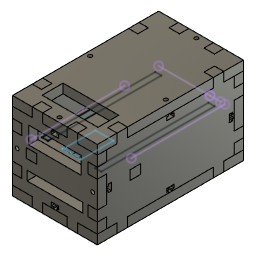
Basic-Case (Autodesk Fusion 360 design; units mm, degrees)
Autodesk Fusion 360 part; units mm, degrees
(part 1 of 2)
ref_plane "WorkPlane4" through (0, 29.5, 0) normal (0, 1, 0) x (0, 0, 1)
ref_plane "WorkPlane5" through (0, 0, 27.5) normal (0, 0, 1) x (1, 0, 0)
ref_plane "WorkPlane9" through (0, 0, -27.5) normal (0, 0, 1) x (1, 0, 0)
ref_plane "WorkPlane11" through (-14.285, 0, 0) normal (1, 0, 0) x (0, 1, 0)
ref_plane "WorkPlane12" through (14.285, 0, 0) normal (1, 0, 0) x (0, 1, 0)
sketch "Sketch1" plane through (0, 0, 0) normal (0, 1, 0) x (1, 0, 0)
  line L0 (12.785, -26) -> (-12.785, -26) construction
  line L1 (-12.785, -26) -> (-12.785, 26) construction
  line L2 (-12.785, 26) -> (12.785, 26) construction
  line L3 (12.785, 26) -> (12.785, -26) construction
  line L4 (12.785, -26) -> (-12.785, 26) construction
  line L5 (-12.785, -26) -> (12.785, 26) construction
  line L6 (-14.285, -27.5) -> (-14.285, 27.5)
  line L7 (-14.285, 27.5) -> (14.285, 27.5)
  line L8 (14.285, 27.5) -> (14.285, -27.5)
  line L9 (14.285, -27.5) -> (-14.285, -27.5)
  line L10 (-18.285, -31.5) -> (-18.285, 31.5)
  line L11 (-18.285, 31.5) -> (18.285, 31.5)
  line L12 (18.285, 31.5) -> (18.285, -31.5)
  line L13 (18.285, -31.5) -> (-18.285, -31.5)
  line L14 (-18.285, -23) -> (-12.785, -23)
  line L15 (-18.285, -18.5) -> (-14.285, -18.5)
  line L16 (-9.785, -27.5) -> (-9.785, -31.5)
  line L17 (-5.285, -31.5) -> (-5.285, -27.5)
  line L18 (5.285, -27.5) -> (5.285, -31.5)
  line L19 (9.785, -31.5) -> (9.785, -27.5)
  line L20 (14.285, -23) -> (18.285, -23)
  line L21 (14.285, -18.5) -> (18.285, -18.5)
  line L22 (14.285, 23) -> (18.285, 23)
  line L23 (18.285, 18.5) -> (14.285, 18.5)
  line L24 (9.785, 31.5) -> (9.785, 27.5)
  line L25 (5.285, 31.5) -> (5.285, 27.5)
  line L26 (-9.785, 31.5) -> (-9.785, 27.5)
  line L27 (-5.285, 27.5) -> (-5.285, 31.5)
  line L28 (-14.285, 23) -> (-18.285, 23)
  line L29 (-18.285, 18.5) -> (-14.285, 18.5)
  line L30 (0, -27.5) -> (0, -31.5) construction
  line L31 (14.285, 0) -> (18.285, 0) construction
  line L32 (-18.285, 0) -> (-14.285, 0) construction
  line L33 (0, 31.5) -> (0, 27.5) construction
  circle A0 centre (16.285, 0) radius 0.8
  circle A1 centre (0, 29.5) radius 0.8
  circle A2 centre (-16.285, 0) radius 0.8
  circle A3 centre (0, -29.5) radius 0.8
  dimension "d1" = 52
  dimension "d2" = 25.57
  dimension "d3" = 1.5
  dimension "d4" = 5.5
  dimension "d385" = 4.5
  dimension "d386" = 4.5
  dimension "d387" = 4.5
  dimension "d388" = 4.5
  dimension "d389" = 4.5
  dimension "d391" = 4.5
  dimension "d392" = 4.5
  dimension "d394" = 4.5
  dimension "d395" = 4.5
  dimension "d396" = 4.5
  dimension "d397" = 4.5
  dimension "d399" = 4.5
  dimension "d402" = 1.6
  dimension "d403" = 1.6
  dimension "d404" = 1.6
  dimension "d405" = 1.6
  dimension "d437" = 4.5
  dimension "d438" = 4.5
  dimension "d439" = 4.5
  dimension "d440" = 4.5
  constraint perpendicular L0 L1
  constraint parallel L0 L2
  constraint parallel L1 L3
  constraint horizontal L0
  constraint coincident L4 origin
  constraint coincident L5 origin
  constraint coincident L10 L14.start
  constraint coincident L1 L14.end
  constraint perpendicular L6 L14
  constraint coincident L10 L15.start
  constraint coincident L6 L15.end
  constraint perpendicular L1 L15
  constraint coincident L9 L16.start
  constraint coincident L13 L16.end
  constraint perpendicular L13 L16
  constraint coincident L13 L17.start
  constraint coincident L9 L17.end
  constraint perpendicular L9 L17
  constraint coincident L9 L18.start
  constraint coincident L13 L18.end
  constraint perpendicular L13 L18
  constraint coincident L13 L19.start
  constraint coincident L9 L19.end
  constraint perpendicular L0 L19
  constraint coincident L8 L20.start
  constraint coincident L12 L20.end
  constraint perpendicular L12 L20
  constraint coincident L8 L21.start
  constraint coincident L12 L21.end
  constraint perpendicular L12 L21
  constraint coincident L8 L22.start
  constraint coincident L12 L22.end
  constraint perpendicular L12 L22
  constraint coincident L12 L23.start
  constraint coincident L8 L23.end
  constraint perpendicular L8 L23
  constraint coincident L11 L24.start
  constraint coincident L7 L24.end
  constraint perpendicular L7 L24
  constraint coincident L11 L25.start
  constraint coincident L7 L25.end
  constraint perpendicular L11 L25
  constraint coincident L11 L26.start
  constraint coincident L7 L26.end
  constraint perpendicular L7 L26
  constraint coincident L7 L27.start
  constraint coincident L11 L27.end
  constraint perpendicular L11 L27
  constraint coincident L6 L28.start
  constraint coincident L10 L28.end
  constraint perpendicular L10 L28
  constraint coincident L10 L29.start
  constraint coincident L6 L29.end
  constraint perpendicular L6 L29
  constraint midpoint L9 L30.start
  constraint midpoint L13 L30.end
  constraint midpoint L8 L31.start
  constraint midpoint L12 L31.end
  constraint midpoint L10 L32.start
  constraint midpoint L6 L32.end
  constraint midpoint L11 L33.start
  constraint midpoint L7 L33.end
  constraint midpoint L31 A0.centre
  constraint midpoint L33 A1.centre
  constraint midpoint L32 A2.centre
  constraint midpoint L30 A3.centre
  measures "d1" distance of L0.start L2.end
  measures "d2" distance of L0.start L0.end
  measures "d385" distance of L28 L29
  measures "d386" distance of L26 L27
  measures "d387" distance of L6.end L26
  measures "d388" distance of L24 L25
  measures "d389" distance of L7.end L24
  measures "d391" distance of L22 L23
  measures "d392" distance of L20 L21
  measures "d394" distance of L8.end L19
  measures "d395" distance of L18 L19
  measures "d396" distance of L6.start L16
  measures "d397" distance of L16 L17
  measures "d399" distance of L14 L15
  measures "d402" diameter of A3
  measures "d403" diameter of A0
  measures "d404" diameter of A2
  measures "d405" diameter of A1
  measures "d437" distance of L6.start L14
  measures "d438" distance of L6.end L28
  measures "d439" distance of L7.end L22
  measures "d440" distance of L8.end L20
sketch "Sketch33" plane through (0, 29.5, 0) normal (0, 1, 0) x (1, 0, 0)
  line L0 (-18.285, 31.5) -> (18.285, 31.5)
  line L1 (-18.285, -31.5) -> (-18.285, 31.5)
  line L2 (18.285, -31.5) -> (-18.285, -31.5)
  line L3 (-14.285, -27.5) -> (-14.285, 27.5)
  line L4 (-14.285, 27.5) -> (14.285, 27.5)
  line L5 (-14.285, 23) -> (-18.285, 23)
  line L6 (-18.285, 18.5) -> (-14.285, 18.5)
  line L7 (-9.785, 31.5) -> (-9.785, 27.5)
  line L8 (-5.285, 27.5) -> (-5.285, 31.5)
  line L9 (5.285, 31.5) -> (5.285, 27.5)
  line L10 (9.785, 31.5) -> (9.785, 27.5)
  line L11 (14.285, 27.5) -> (14.285, -27.5)
  line L12 (14.285, 23) -> (18.285, 23)
  line L13 (18.285, 18.5) -> (14.285, 18.5)
  line L14 (18.285, 31.5) -> (18.285, -31.5)
  line L15 (14.285, -18.5) -> (18.285, -18.5)
  line L16 (14.285, -23) -> (18.285, -23)
  line L17 (9.785, -31.5) -> (9.785, -27.5)
  line L18 (5.285, -27.5) -> (5.285, -31.5)
  line L19 (-5.285, -31.5) -> (-5.285, -27.5)
  line L20 (-9.785, -27.5) -> (-9.785, -31.5)
  line L21 (-18.285, -23) -> (-12.785, -23)
  line L22 (-18.285, -18.5) -> (-14.285, -18.5)
  line L23 (14.285, -27.5) -> (-14.285, -27.5)
  circle A0 centre (0, -29.5) radius 0.8
  circle A1 centre (0, 29.5) radius 0.8
  circle A2 centre (-16.285, 0) radius 0.8
  circle A3 centre (16.285, 0) radius 0.8
  point P0 (16.285, 0)
  point P1 (-16.285, 0)
sketch "Sketch24" plane through (0, 0, 27.5) normal (0, 0, 1) x (1, 0, 0)
  line L0 (18.285, 0) -> (-18.285, 0)
  line L1 (18.285, 29.5) -> (-18.285, 29.5)
  line L2 (-9.785, 29.5) -> (-9.785, 33.5)
  line L3 (-5.285, 29.5) -> (-5.285, 33.5)
  line L4 (5.285, 29.5) -> (5.285, 33.5)
  line L5 (9.785, 29.5) -> (9.785, 33.5)
  line L6 (-9.785, 0) -> (-9.785, -4)
  line L7 (-5.285, 0) -> (-5.285, -4)
  line L8 (5.285, 0) -> (5.285, -4)
  line L9 (9.785, 0) -> (9.785, -4)
  line L10 (-0.8, 29.5) -> (-0.8, 28.8)
  line L11 (-0.8, 28.8) -> (-1.6, 28.8)
  line L12 (-1.6, 28.8) -> (-1.6, 27.4)
  line L13 (-1.6, 27.4) -> (1.6, 27.4)
  line L14 (1.6, 27.4) -> (1.6, 28.8)
  line L15 (1.6, 28.8) -> (0.8, 28.8)
  line L16 (0.8, 28.8) -> (0.8, 29.5)
  line L17 (-0.8, 0) -> (-0.8, 0.7)
  line L18 (-1.6, 0.7) -> (-1.6, 2.1)
  line L19 (-1.6, 2.1) -> (1.6, 2.1)
  line L20 (-0.8, 0.7) -> (-1.6, 0.7)
  line L21 (1.6, 0.7) -> (0.8, 0.7)
  line L22 (0.8, 0.7) -> (0.8, 0)
  line L23 (1.6, 2.1) -> (1.6, 0.7)
  line L24 (0, 27.4) -> (0, 29.5) construction
  line L25 (0, 2.1) -> (0, 0) construction
  line L26 (14.285, 25) -> (24.3607, 25)
  line L27 (14.285, 4.5) -> (18.285, 4.5)
  line L28 (-14.285, 20.5) -> (-18.285, 20.5)
  line L29 (-18.285, 9) -> (-14.285, 9)
  line L30 (-18.285, 33.5) -> (-18.285, -4)
  line L31 (-18.285, -4) -> (18.285, -4)
  line L32 (18.285, -4) -> (18.285, 33.5)
  line L33 (18.285, 33.5) -> (-18.285, 33.5)
  line L34 (-14.285, 29.5) -> (-14.285, 0)
  line L35 (14.285, 29.5) -> (14.285, 0)
  line L36 (18.285, 9) -> (14.285, 9)
  line L37 (18.285, 20.5) -> (14.285, 20.5)
  line L38 (-14.285, 25) -> (-18.285, 25)
  line L39 (-14.285, 4.5) -> (-18.285, 4.5)
  line L40 (18.285, 14.75) -> (14.285, 14.75) construction
  line L41 (-14.285, 14.75) -> (-14.285, 14.6467)
  line L42 (-18.285, 14.75) -> (-14.285, 14.75) construction
  circle A0 centre (16.285, 14.75) radius 0.8
  circle A1 centre (-16.285, 14.75) radius 0.8
  line L43 (0, 0) -> (0, 33.5) construction
  point P0 (-5.285, 0)
  point P1 (-9.785, 0)
  point P2 (5.285, 0)
  point P3 (9.785, 0)
  point P4 (0, 29.5)
  point P5 (-9.785, 29.5)
  point P6 (-5.285, 29.5)
  point P7 (9.785, 29.5)
  point P8 (5.285, 29.5)
  dimension "d406" = 3.2
  dimension "d407" = 1.4
  dimension "d409" = 1.6
  dimension "d410" = 1.6
  dimension "d411" = 3.2
  dimension "d413" = 1.4
  dimension "d420" = 6.1
  dimension "d421" = 4
  dimension "d422" = 4
  dimension "d424" = 6.1
  dimension "d425" = 4
  dimension "d426" = 4
  dimension "d427" = 4.5
  dimension "d428" = 4.5
  dimension "d429" = 4.5
  dimension "d430" = 4.5
  dimension "d433" = 4.5
  dimension "d434" = 4.5
  dimension "d435" = 1.6
  dimension "d436" = 1.6
  dimension "d482" = 4.5
  dimension "d483" = 4.5
  constraint coincident P1 L6.start
  constraint coincident P0 L7.start
  constraint coincident P2 L8.start
  constraint perpendicular L0 L8
  constraint coincident P3 L9.start
  constraint perpendicular L10 L11
  constraint perpendicular L12 L13
  constraint perpendicular L14 L15
  constraint collinear L11 L15
  constraint equal L11 L15
  constraint equal L17 L22
  constraint equal L18 L23
  constraint equal L20 L21
  constraint perpendicular L18 L19
  constraint perpendicular L19 L23
  constraint perpendicular L18 L20
  constraint perpendicular L21 L22
  constraint midpoint L13 L24.start
  constraint coincident P4 L24.end
  constraint perpendicular L1 L24
  constraint midpoint L19 L25.start
  constraint coincident L25.end L43.start
  constraint perpendicular L0 L25
  constraint perpendicular L1 L3
  constraint perpendicular L1 L2
  constraint perpendicular L1 L4
  constraint perpendicular L1 L5
  constraint vertical L30
  constraint perpendicular L32 L33
  constraint perpendicular L30 L33
  constraint perpendicular L30 L31
  constraint coincident L2.end L33
  constraint coincident L3.end L33
  constraint coincident L4.end L33
  constraint coincident L5.end L33
  constraint coincident L1.start L32
  constraint coincident L1.end L30
  constraint coincident L6.end L31
  constraint coincident L7.end L31
  constraint coincident L0 L17.start
  constraint coincident L0 L22.end
  constraint coincident L1 L10.start
  constraint coincident L1 L16.end
  constraint coincident L8.end L31
  constraint coincident L9.end L31
  constraint coincident L1 L34.start
  constraint coincident L0 L34.end
  constraint perpendicular L0 L34
  constraint coincident L1 L35.start
  constraint coincident L0 L35.end
  constraint perpendicular L0 L35
  constraint coincident L28.start L34
  constraint coincident L29.end L34
  constraint coincident L26.start L35
  constraint coincident L27.start L35
  constraint perpendicular L0 L9
  constraint perpendicular L0 L6
  constraint perpendicular L0 L7
  constraint coincident L27.end L32
  constraint perpendicular L27 L32
  constraint coincident L32 L36.start
  constraint coincident L35 L36.end
  constraint perpendicular L35 L36
  constraint coincident L32 L37.start
  constraint coincident L35 L37.end
  constraint perpendicular L35 L37
  constraint coincident L34 L38.start
  constraint coincident L30 L38.end
  constraint perpendicular L30 L38
  constraint coincident L34 L39.start
  constraint coincident L30 L39.end
  constraint perpendicular L30 L39
  constraint coincident L29.start L30
  constraint perpendicular L29 L30
  constraint midpoint L32 L40.start
  constraint midpoint L35 L40.end
  constraint midpoint L34 L41.start
  constraint coincident L34 L41.end
  constraint parallel L34 L41
  constraint midpoint L30 L42.start
  constraint midpoint L40 A0.centre
  constraint midpoint L42 A1.centre
  constraint midpoint L33 L43.end
  constraint vertical L43
  constraint equal L12 L14
  constraint coincident L1 P8
  constraint coincident L1 P7
  constraint coincident L1 P6
  constraint coincident L1 P5
  constraint coincident P5 L2.start
  constraint coincident P6 L3.start
  constraint coincident P7 L5.start
  constraint coincident P8 L4.start
  constraint coincident L0.end L30
  constraint coincident L28.end L30
  measures "d406" distance of L12.end L13.end
  measures "d407" distance of L13.end L14.end
  measures "d409" distance of L10 L16
  measures "d410" distance of L17 L22
  measures "d411" horizontal distance of L18.end L19.end
  measures "d413" distance of L18.start L18.end
  measures "d420" distance of L13 L33
  measures "d421" distance of L1 L33
  measures "d422" distance of L0 L31
  measures "d424" distance of L19 L31
  measures "d425" distance of L30 L34
  measures "d426" distance of L32 L35
  measures "d427" distance of L28 L38
  measures "d428" distance of L29 L39
  measures "d429" distance of L26 L37
  measures "d430" distance of L27 L36
  measures "d433" distance of L0 L39
  measures "d434" distance of L0.start L27
  measures "d435" diameter of A1
  measures "d436" diameter of A0
  measures "d482" distance of L1 L38
  measures "d483" distance of L1 L26
sketch "Sketch38" plane through (0, 0, -27.5) normal (0, 0, 1) x (1, 0, 0)
  line L0 (18.285, 33.5) -> (-18.285, 33.5)
  line L1 (18.285, -4) -> (18.285, 33.5)
  line L2 (14.285, 29.5) -> (14.285, 0)
  line L3 (18.285, 29.5) -> (-18.285, 29.5)
  line L4 (9.785, 29.5) -> (9.785, 33.5)
  line L5 (5.285, 29.5) -> (5.285, 33.5)
  line L6 (-5.285, 29.5) -> (-5.285, 33.5)
  line L7 (-9.785, 29.5) -> (-9.785, 33.5)
  line L8 (0.8, 28.8) -> (0.8, 29.5)
  line L9 (1.6, 28.8) -> (0.8, 28.8)
  line L10 (1.6, 27.4) -> (1.6, 28.8)
  line L11 (-1.6, 27.4) -> (1.6, 27.4)
  line L12 (-1.6, 28.8) -> (-1.6, 27.4)
  line L13 (-0.8, 28.8) -> (-1.6, 28.8)
  line L14 (-0.8, 29.5) -> (-0.8, 28.8)
  line L15 (-14.285, 29.5) -> (-14.285, 0)
  line L16 (-18.285, 33.5) -> (-18.285, -4)
  line L17 (-14.285, 25) -> (-18.285, 25)
  line L18 (-14.285, 20.5) -> (-18.285, 20.5)
  circle A0 centre (-16.285, 14.75) radius 0.8
  line L19 (-18.285, 9) -> (-14.285, 9)
  line L20 (-14.285, 4.5) -> (-18.285, 4.5)
  line L21 (18.285, 0) -> (-18.285, 0)
  line L22 (-9.785, 0) -> (-9.785, -4)
  line L23 (-18.285, -4) -> (18.285, -4)
  line L24 (-5.285, 0) -> (-5.285, -4)
  line L25 (9.785, 0) -> (9.785, -4)
  line L26 (5.285, 0) -> (5.285, -4)
  line L27 (14.285, 4.5) -> (18.285, 4.5)
  line L28 (18.285, 9) -> (14.285, 9)
  circle A1 centre (16.285, 14.75) radius 0.8
  line L29 (18.285, 20.5) -> (14.285, 20.5)
  line L30 (14.285, 25) -> (24.3607, 25)
  line L31 (-1.6, 2.1) -> (1.6, 2.1)
  line L32 (1.6, 2.1) -> (1.6, 0.7)
  line L33 (1.6, 0.7) -> (0.8, 0.7)
  line L34 (-0.8, 0.7) -> (-1.6, 0.7)
  line L35 (-0.8, 0) -> (-0.8, 0.7)
  line L36 (0.8, 0.7) -> (0.8, 0)
  line L37 (-1.6, 0.7) -> (-1.6, 2.1)
sketch "Sketch39" plane through (14.285, 0, 0) normal (1, 0, 0) x (0, 1, 0)
  line L0 (29.5, -31.5) -> (29.5, 31.5)
  line L1 (0, -31.5) -> (0, 31.5)
  line L2 (-4, 27.5) -> (33.5, 27.5)
  line L3 (-4, -27.5) -> (33.5, -27.5)
  line L4 (33.5, 31.5) -> (33.5, -31.5)
  line L5 (33.5, -31.5) -> (-4, -31.5)
  line L6 (-4, -31.5) -> (-4, 31.5)
  line L7 (-4, 31.5) -> (33.5, 31.5)
  line L8 (29.5, 23) -> (33.5, 23)
  line L9 (29.5, 18.5) -> (33.5, 18.5)
  line L10 (29.5, -18.5) -> (33.5, -18.5)
  line L11 (29.5, -23) -> (33.5, -23)
  line L12 (25, -27.5) -> (25, -31.5)
  line L13 (20.5, -27.5) -> (20.5, -31.5)
  line L14 (9, -27.5) -> (9, -31.5)
  line L15 (4.5, -27.5) -> (4.5, -31.5)
  line L16 (0, -18.5) -> (-4, -18.5)
  line L17 (0, -23) -> (-4, -23)
  line L18 (0, 23) -> (-4, 23)
  line L19 (0, 18.5) -> (-4, 18.5)
  line L20 (25, 27.5) -> (25, 31.5)
  line L21 (20.5, 27.5) -> (20.5, 31.5)
  line L22 (9, 27.5) -> (9, 31.5)
  line L23 (4.5, 27.5) -> (4.5, 31.5)
  line L24 (29.5, 0.8) -> (28.8, 0.8)
  line L25 (28.8, 0.8) -> (28.8, 1.6)
  line L26 (27.4, 1.6) -> (27.4, -1.6)
  line L27 (27.4, -1.6) -> (28.8, -1.6)
  line L28 (28.8, -1.6) -> (28.8, -0.8)
  line L29 (28.8, -0.8) -> (29.5, -0.8)
  line L30 (15.55, -27.5) -> (15.55, -26.8)
  line L31 (15.55, -26.8) -> (16.35, -26.8)
  line L32 (16.35, -26.8) -> (16.35, -25.4)
  line L33 (16.35, -25.4) -> (13.15, -25.4)
  line L34 (13.15, -25.4) -> (13.15, -26.8)
  line L35 (13.15, -26.8) -> (13.95, -26.8)
  line L36 (13.95, -26.8) -> (13.95, -27.5)
  line L37 (0, 0.8) -> (0.7, 0.8)
  line L38 (0.7, 0.8) -> (0.7, 1.6)
  line L39 (0.7, 1.6) -> (2.1, 1.6)
  line L40 (2.1, 1.6) -> (2.1, -1.6)
  line L41 (2.1, -1.6) -> (0.7, -1.6)
  line L42 (0.7, -1.6) -> (0.7, -0.8)
  line L43 (0.7, -0.8) -> (0, -0.8)
  line L44 (13.95, 27.5) -> (13.95, 26.8)
  line L45 (13.95, 26.8) -> (13.15, 26.8)
  line L46 (13.15, 26.8) -> (13.15, 25.4)
  line L47 (13.15, 25.4) -> (16.35, 25.4)
  line L48 (16.35, 25.4) -> (16.35, 26.8)
  line L49 (16.35, 26.8) -> (15.55, 26.8)
  line L50 (15.55, 26.8) -> (15.55, 27.5)
  line L51 (14.75, 27.5) -> (14.75, 25.4) construction
  line L52 (33.5, 0) -> (27.4, 0) construction
  line L53 (14.75, -25.4) -> (14.75, -31.5) construction
  line L54 (-4, 0) -> (2.1, 0) construction
  line L55 (28.8, 1.6) -> (27.4, 1.6)
  point P0 (29.5, 23)
  point P1 (29.5, 18.5)
  point P2 (29.5, -18.5)
  point P3 (29.5, -23)
  point P4 (0, -23)
  point P5 (0, 18.5)
  point P6 (29.5, 0)
  point P7 (0, -18.5)
  point P8 (0, 23)
  point P9 (9, 27.5)
  point P10 (4.5, 27.5)
  point P11 (25, 27.5)
  point P12 (20.5, 27.5)
  point P13 (29.5, 27.5)
  point P14 (25, -27.5)
  point P15 (20.5, -27.5)
  point P16 (9, -27.5)
  point P17 (4.5, -27.5)
  point P18 (14.75, -27.5)
  point P19 (14.75, 27.5)
  dimension "d452" = 1.4
  dimension "d453" = 3.2
  dimension "d454" = 1.6
  dimension "d455" = 6.1
  dimension "d456" = 3.2
  dimension "d457" = 1.6
  dimension "d458" = 1.4
  dimension "d459" = 6.1
  dimension "d460" = 1.6
  dimension "d461" = 3.2
  dimension "d462" = 1.4
  dimension "d463" = 6.1
  dimension "d464" = 1.4
  dimension "d465" = 1.6
  dimension "d466" = 3.2
  dimension "d467" = 6.1
  constraint perpendicular L2 L4
  constraint perpendicular L4 L5
  constraint perpendicular L5 L6
  constraint coincident L2.end L4
  constraint coincident L0.end L7
  constraint coincident L1.end L7
  constraint coincident L2.start L6
  constraint coincident L1.start L5
  constraint coincident P0 L8.start
  constraint coincident L4 L8.end
  constraint perpendicular L4 L8
  constraint coincident P1 L9.start
  constraint coincident L4 L9.end
  constraint perpendicular L4 L9
  constraint coincident P2 L10.start
  constraint coincident L4 L10.end
  constraint perpendicular L4 L10
  constraint coincident P3 L11.start
  constraint coincident L4 L11.end
  constraint perpendicular L4 L11
  constraint coincident P14 L12.start
  constraint coincident L5 L12.end
  constraint perpendicular L5 L12
  constraint coincident P15 L13.start
  constraint coincident L5 L13.end
  constraint perpendicular L5 L13
  constraint coincident P16 L14.start
  constraint coincident L5 L14.end
  constraint perpendicular L5 L14
  constraint coincident P17 L15.start
  constraint coincident L5 L15.end
  constraint perpendicular L5 L15
  constraint coincident P7 L16.start
  constraint coincident L6 L16.end
  constraint perpendicular L6 L16
  constraint coincident P4 L17.start
  constraint coincident L6 L17.end
  constraint perpendicular L6 L17
  constraint coincident P8 L18.start
  constraint coincident L6 L18.end
  constraint perpendicular L6 L18
  constraint coincident P5 L19.start
  constraint coincident L6 L19.end
  constraint perpendicular L6 L19
  constraint coincident P11 L20.start
  constraint coincident L7 L20.end
  constraint perpendicular L7 L20
  constraint coincident P12 L21.start
  constraint coincident L7 L21.end
  constraint perpendicular L7 L21
  constraint coincident P9 L22.start
  constraint coincident L7 L22.end
  constraint perpendicular L7 L22
  constraint coincident P10 L23.start
  constraint coincident L7 L23.end
  constraint perpendicular L7 L23
  constraint coincident L0 L24.start
  constraint perpendicular L0 L24
  constraint perpendicular L24 L25
  constraint perpendicular L26 L27
  constraint perpendicular L27 L28
  constraint coincident L0 L29.end
  constraint perpendicular L0 L29
  constraint coincident L3 L30.start
  constraint perpendicular L3 L30
  constraint perpendicular L30 L31
  constraint perpendicular L3 L32
  constraint perpendicular L32 L33
  constraint perpendicular L33 L34
  constraint perpendicular L32 L35
  constraint coincident L3 L36.end
  constraint perpendicular L3 L36
  constraint coincident L1 L37.start
  constraint perpendicular L1 L37
  constraint perpendicular L37 L38
  constraint perpendicular L38 L39
  constraint perpendicular L39 L40
  constraint perpendicular L38 L41
  constraint perpendicular L39 L42
  constraint coincident L1 L43.end
  constraint perpendicular L1 L43
  constraint coincident L2 L44.start
  constraint perpendicular L2 L44
  constraint perpendicular L44 L45
  constraint perpendicular L2 L46
  constraint perpendicular L44 L47
  constraint perpendicular L47 L48
  constraint perpendicular L48 L49
  constraint coincident L2 L50.end
  constraint perpendicular L2 L50
  constraint coincident P19 L51.start
  constraint midpoint L47 L51.end
  constraint midpoint L4 L52.start
  constraint midpoint L26 L52.end
  constraint midpoint L33 L53.start
  constraint midpoint L5 L53.end
  constraint midpoint L6 L54.start
  constraint midpoint L40 L54.end
  constraint vertical L53
  constraint horizontal L52
  constraint vertical L51
  constraint horizontal L54
  constraint equal L38 L42
  constraint equal L37 L43
  constraint equal L24 L29
  constraint equal L25 L28
  constraint equal L44 L50
  constraint equal L45 L49
  constraint equal L31 L35
  constraint equal L30 L36
  constraint perpendicular L26 L55
  constraint vertical L26
  measures "d452" distance of L31.end L32.end
  measures "d453" distance of L32.end L33.end
  measures "d454" distance of L30 L36
  measures "d455" distance of L5 L33
  measures "d456" distance of L26.start L26.end
  measures "d457" distance of L24 L29
  measures "d458" distance of L26.end L27.end
  measures "d459" distance of L4 L26
  measures "d460" distance of L44 L50
  measures "d461" distance of L46.end L47.end
  measures "d462" distance of L47.end L48.end
  measures "d463" distance of L7 L47
  measures "d464" distance of L38.end L39.end
  measures "d465" distance of L37 L43
  measures "d466" distance of L39.end L40.end
  measures "d467" distance of L6 L40
sketch "Sketch40" plane through (-14.285, 0, 0) normal (1, 0, 0) x (0, 1, 0)
  line L0 (33.5, 31.5) -> (33.5, -31.5)
  line L1 (33.5, -31.5) -> (-4, -31.5)
  line L2 (-4, -27.5) -> (33.5, -27.5)
  line L3 (29.5, -31.5) -> (29.5, 31.5)
  line L4 (29.5, -23) -> (33.5, -23)
  line L5 (29.5, -18.5) -> (33.5, -18.5)
  line L6 (25, -27.5) -> (25, -31.5)
  line L7 (20.5, -27.5) -> (20.5, -31.5)
  line L8 (9, -27.5) -> (9, -31.5)
  line L9 (4.5, -27.5) -> (4.5, -31.5)
  line L10 (-4, -31.5) -> (-4, 31.5)
  line L11 (0, -31.5) -> (0, 31.5)
  line L12 (0, -23) -> (-4, -23)
  line L13 (0, -18.5) -> (-4, -18.5)
  line L14 (0, 18.5) -> (-4, 18.5)
  line L15 (0, 23) -> (-4, 23)
  line L16 (-4, 27.5) -> (33.5, 27.5)
  line L17 (9, 27.5) -> (9, 31.5)
  line L18 (4.5, 27.5) -> (4.5, 31.5)
  line L19 (20.5, 27.5) -> (20.5, 31.5)
  line L20 (25, 27.5) -> (25, 31.5)
  line L21 (29.5, 18.5) -> (33.5, 18.5)
  line L22 (29.5, 23) -> (33.5, 23)
  line L23 (28.8, -0.8) -> (29.5, -0.8)
  line L24 (28.8, -1.6) -> (28.8, -0.8)
  line L25 (27.4, -1.6) -> (28.8, -1.6)
  line L26 (27.4, 1.6) -> (27.4, -1.6)
  line L27 (28.8, 1.6) -> (27.4, 1.6)
  line L28 (28.8, 0.8) -> (28.8, 1.6)
  line L29 (29.5, 0.8) -> (28.8, 0.8)
  line L30 (15.55, -27.5) -> (15.55, -26.8)
  line L31 (16.35, -26.8) -> (16.35, -25.4)
  line L32 (16.35, -25.4) -> (13.15, -25.4)
  line L33 (15.55, -26.8) -> (16.35, -26.8)
  line L34 (13.15, -25.4) -> (13.15, -26.8)
  line L35 (13.15, -26.8) -> (13.95, -26.8)
  line L36 (13.95, -26.8) -> (13.95, -27.5)
  line L37 (2.1, -1.6) -> (0.7, -1.6)
  line L38 (2.1, 1.6) -> (2.1, -1.6)
  line L39 (0.7, 1.6) -> (2.1, 1.6)
  line L40 (0.7, 0.8) -> (0.7, 1.6)
  line L41 (0, 0.8) -> (0.7, 0.8)
  line L42 (0.7, -0.8) -> (0, -0.8)
  line L43 (0.7, -1.6) -> (0.7, -0.8)
  line L44 (13.15, 25.4) -> (16.35, 25.4)
  line L45 (16.35, 25.4) -> (16.35, 26.8)
  line L46 (16.35, 26.8) -> (15.55, 26.8)
  line L47 (15.55, 26.8) -> (15.55, 27.5)
  line L48 (13.95, 27.5) -> (13.95, 26.8)
  line L49 (13.95, 26.8) -> (13.15, 26.8)
  line L50 (13.15, 26.8) -> (13.15, 25.4)
  line L51 (-4, 31.5) -> (33.5, 31.5)
extrude "Extrude52" add sketch "Sketch1" against normal blind 4 contours L6 L10 L15 L29 | L6 L7 L8 L9 | L6 L9 L10 L13 L14 L16 | L6 L7 L10 L11 L26 L28 | L9 L13 L17 L18 | L7 L11 L25 L27 | L8 L9 L12 L13 L19 L20 | L7 L8 L11 L12 L22 L24 | L8 L12 L21 L23 makes body 1
extrude "Extrude53" add sketch "Sketch33" along normal blind 4 separate body contours L0 L1 L3 L4 L5 L7 | L0 L4 L8 L9 | L3 L4 L11 L23 | L1 L3 L6 L22 | L0 L4 L10 L11 L12 L14 | L1 L2 L3 L20 L21 L23 | L11 L13 L14 L15 | L2 L18 L19 L23 | L2 L11 L14 L16 L17 L23 makes body 2
extrude "Extrude54" add sketch "Sketch24" along normal blind 4 separate body contours L0 L27 L32 L35 | L0 L1 L10 L11 L12 L13 L14 L15 L16 L17 L18 L19 L20 L21 L22 L23 L34 L35 L41 | L0 L8 L9 L31 | L32 L35 L36 L37 | L0 L6 L7 L31 | L1 L26 L32 L35 | L1 L4 L5 L33 | L0 L30 L34 L39 | L28 L29 L30 L34 L41 | L1 L2 L3 L33 | L1 L30 L34 L38 makes body 3
extrude "Extrude55" add sketch "Sketch38" against normal blind 4 separate body contours L0 L3 L4 L5 | L1 L2 L3 L30 | L2 L3 L8 L9 L10 L11 L12 L13 L14 L15 L21 L31 L32 L33 L34 L35 L36 L37 | L0 L3 L6 L7 | L1 L2 L28 L29 | L1 L2 L21 L27 | L3 L15 L16 L17 | L15 L16 L18 L19 | L21 L23 L25 L26 | L15 L16 L20 L21 | L21 L22 L23 L24 makes body 4
extrude "Extrude56" add sketch "Sketch39" along normal blind 4 separate body contours L0 L1 L2 L3 L24 L25 L26 L27 L28 L29 L30 L31 L32 L33 L34 L35 L36 L37 L38 L39 L40 L41 L42 L43 L44 L45 L46 L47 L48 L49 L50 L55 | L0 L4 L10 L11 | L3 L5 L12 L13 | L0 L4 L8 L9 | L3 L5 L14 L15 | L2 L7 L20 L21 | L1 L6 L16 L17 | L2 L7 L22 L23 | L1 L6 L18 L19 makes body 5
extrude "Extrude57" add sketch "Sketch40" against normal blind 4 separate body contours L0 L3 L21 L22 | L2 L3 L11 L16 L23 L24 L25 L26 L27 L28 L29 L30 L31 L32 L33 L34 L35 L36 L37 L38 L39 L40 L41 L42 L43 L44 L45 L46 L47 L48 L49 L50 | L16 L19 L20 L51 | L0 L3 L4 L5 | L16 L17 L18 L51 | L1 L2 L6 L7 | L10 L11 L14 L15 | L1 L2 L8 L9 | L10 L11 L12 L13 makes body 6
ref_plane "WorkPlane13" through (0, 13, 0) normal (0, 1, 0) x (0, 0, 1)
sketch "Sketch41" plane through (0, 13, 0) normal (0, 1, 0) x (1, 0, 0)
  line L0 (-14.285, -27.5) -> (-14.285, 27.5)
  line L1 (-14.285, 27.5) -> (14.285, 27.5)
  line L2 (14.285, 27.5) -> (14.285, -27.5)
  line L3 (14.285, -27.5) -> (-14.285, -27.5)
  line L4 (-18.285, -18.5) -> (-14.285, -18.5) construction
  line L5 (18.285, 31.5) -> (18.285, -31.5)
  line L6 (-18.285, 31.5) -> (18.285, 31.5)
  line L7 (-18.285, -31.5) -> (-18.285, 31.5)
  line L8 (18.285, -31.5) -> (-18.285, -31.5)
  line L9 (-18.285, 17.35) -> (-14.285, 17.35)
  line L10 (-18.285, 12.85) -> (-14.285, 12.85)
  line L11 (7.85, 27.5) -> (7.85, 31.5)
  line L12 (12.35, 27.5) -> (12.35, 31.5)
  line L13 (14.285, -12.85) -> (18.285, -12.85)
  line L14 (14.285, -17.35) -> (18.285, -17.35)
  line L15 (-7.85, -27.5) -> (-7.85, -31.5)
  line L16 (-12.35, -27.5) -> (-12.35, -31.5)
  circle A0 centre (0, 29.5) radius 0.8 construction
  circle A1 centre (16.285, 0) radius 0.8 construction
  circle A2 centre (-16.285, 0) radius 0.8 construction
  circle A3 centre (0, -29.5) radius 0.8 construction
  line L17 (-12.35, -27.5) -> (-7.85, -31.5) construction
  line L18 (14.285, -17.35) -> (18.285, -12.85) construction
  line L19 (7.85, 31.5) -> (12.35, 27.5) construction
  line L20 (-18.285, 17.35) -> (-14.285, 12.85) construction
  line L21 (-20.2, -29.5) -> (0, -29.5) construction
  line L22 (16.285, -30.2) -> (16.285, 0) construction
  line L23 (-16.285, 0) -> (-16.285, 30.2) construction
  line L24 (0, 29.5) -> (20.2, 29.5) construction
  line L25 (14.285, 27.5) -> (14.285, 31.5) construction
  line L26 (-14.285, 27.5) -> (-18.285, 27.5) construction
  line L27 (-14.285, -27.5) -> (-14.285, -31.5) construction
  line L28 (14.285, -27.5) -> (18.285, -27.5) construction
  point P0 (0, -29.5)
  dimension "d474" = 4.5
  dimension "d475" = 4.5
  dimension "d476" = 4.5
  dimension "d477" = 4.5
  constraint coincident L7 L9.start
  constraint coincident L0 L9.end
  constraint perpendicular L0 L9
  constraint coincident L7 L10.start
  constraint coincident L0 L10.end
  constraint perpendicular L0 L10
  constraint coincident L1 L11.start
  constraint coincident L6 L11.end
  constraint perpendicular L6 L11
  constraint coincident L1 L12.start
  constraint coincident L6 L12.end
  constraint perpendicular L6 L12
  constraint coincident L2 L13.start
  constraint coincident L5 L13.end
  constraint perpendicular L5 L13
  constraint coincident L2 L14.start
  constraint coincident L5 L14.end
  constraint perpendicular L5 L14
  constraint coincident L3 L15.start
  constraint coincident L8 L15.end
  constraint perpendicular L8 L15
  constraint coincident L3 L16.start
  constraint coincident L8 L16.end
  constraint perpendicular L8 L16
  constraint coincident P0 A3.centre
  constraint coincident A1.centre L22.end
  constraint coincident A2.centre L23.start
  constraint coincident A0.centre L24.start
  constraint midpoint L17 L21
  constraint midpoint L18 L22
  constraint midpoint L20 L23
  constraint midpoint L19 L24
  constraint coincident L1.end L2.start
  constraint coincident L6 L25.end
  constraint perpendicular L6 L25
  constraint coincident L0.end L1.start
  constraint coincident L7 L26.end
  constraint perpendicular L7 L26
  constraint coincident L0.start L3.end
  constraint coincident L8 L27.end
  constraint perpendicular L8 L27
  constraint coincident L2.end L3.start
  constraint coincident L5 L28.end
  constraint perpendicular L5 L28
  constraint perpendicular L22 L28
  constraint perpendicular L21 L27
  constraint perpendicular L23 L26
  measures "d474" distance of L9 L10
  measures "d475" distance of L11 L12
  measures "d476" distance of L13 L14
  measures "d477" distance of L15 L16
extrude "Extrude59" cut sketch "Sketch41" along normal blind 4 contours L0 L7 L9 L10 | L3 L8 L15 L16 | L1 L6 L11 L12 | L2 L5 L13 L14 bodies 3 4 5 6
extrude "Extrude58" add sketch "Sketch41" along normal blind 4 separate body contours L0 L1 L2 L3 | L0 L7 L9 L10 | L3 L8 L15 L16 | L1 L6 L11 L12 | L2 L5 L13 L14 makes body 7
ref_plane "WorkPlane15" through (0, 17, 0) normal (0, 1, 0) x (0, 0, 1)
sketch "Sketch45" plane through (0, 17, 0) normal (0, 1, 0) x (1, 0, 0)
  line L0 (12.785, -24.32) -> (10.165, -24.32)
  line L1 (10.165, -24.32) -> (10.165, 24.52)
  line L2 (10.165, 24.52) -> (12.785, 24.52)
  line L3 (12.785, 24.52) -> (12.785, -24.32)
  line L4 (14.285, -12.85) -> (14.285, 27.5)
  line L5 (-12.785, -24.32) -> (-10.165, -24.32)
  line L6 (-10.165, -24.32) -> (-10.165, 24.52)
  line L7 (-10.165, 24.52) -> (-12.785, 24.52)
  line L8 (-12.785, 24.52) -> (-12.785, -24.32)
  line L9 (-14.285, 12.85) -> (-14.285, -27.5)
  line L10 (7.85, 27.5) -> (12.35, 27.5)
  line L11 (7.85, 27.5) -> (-14.285, 27.5)
  line L12 (-3.91, -24.1297) -> (3.89, -24.1297)
  line L13 (3.89, -24.1297) -> (3.89, -10.1297)
  line L14 (3.89, -10.1297) -> (-3.91, -10.1297)
  line L15 (-3.91, -10.1297) -> (-3.91, -24.1297)
  dimension "d489" = 2.62
  dimension "d490" = 48.84
  dimension "d491" = 1.5
  dimension "d492" = 2.62
  dimension "d493" = 48.84
  dimension "d494" = 1.5
  dimension "d496" = 2.98
  dimension "d497" = 2.98
  dimension "d500" = 7.8
  dimension "d501" = 14
  constraint horizontal L0
  constraint vertical L1
  constraint horizontal L2
  constraint vertical L3
  constraint horizontal L5
  constraint vertical L6
  constraint horizontal L7
  constraint vertical L8
  constraint horizontal L12
  constraint vertical L13
  constraint horizontal L14
  constraint vertical L15
  measures "d489" distance of L0.start L0.end
  measures "d490" distance of L0.end L1.end
  measures "d491" distance of L3 L4
  measures "d492" distance of L5.start L5.end
  measures "d493" distance of L5.start L7.end
  measures "d494" distance of L8 L9
  measures "d496" distance of L2 L10
  measures "d497" distance of L7 L11
  measures "d500" distance of L12.start L12.end
  measures "d501" distance of L12.start L14.end
extrude "Extrusion67" cut sketch "Sketch45" against normal blind 33 contours L0 L1 L2 L3 | L5 L6 L7 L8 bodies 1 7
extrude "Extrude61" cut sketch "Sketch45" against normal up to surface (4 mm away) contours L12 L13 L14 L15 bodies 7
ref_plane "Arbeitsebene19" through (0, 0, 0) normal (0, 1, 0) x (1, 0, 0)
sketch "Skizze49" plane through (0, 0, 0) normal (0, 1, 0) x (1, 0, 0)
  line L0 (8.0892, 23.1823) -> (-7.9108, 23.1823)
  line L1 (-7.9108, 23.1823) -> (-7.9108, 14.1817)
  line L2 (-7.9108, 14.1817) -> (8.0892, 14.1817)
  line L3 (8.0892, 14.1817) -> (8.0892, 23.1823)
  dimension "d530" = 16
  constraint horizontal L0
  constraint vertical L1
  constraint horizontal L2
  constraint vertical L3
  measures "d530" distance of L1.end L2.end
extrude "Extrusion65" cut sketch "Skizze49" against normal up to surface (4 mm away) bodies 1
ref_plane "WorkPlane16" through (0, 14.75, 31.5) normal (0, 0, 1) x (1, 0, 0)
sketch "Sketch46" plane through (0, 10.4, 31.5) normal (0, 0, 1) x (1, 0, 0)
  line L0 (-11.285, 8.1) -> (11.285, 8.1)
  line L1 (11.285, 8.1) -> (11.285, 15.5)
  line L2 (11.285, 15.5) -> (-11.285, 15.5)
  line L3 (-11.285, 15.5) -> (-11.285, 8.1)
  line L4 (-14.285, 14.6) -> (-14.285, 10.1)
  line L5 (14.285, 10.1) -> (14.285, 14.6)
  line L6 (1.6, 17) -> (-1.6, 17)
  line L7 (-12.35, 6.6) -> (-7.85, 6.6)
  dimension "d508" = 3
  dimension "d509" = 3
  dimension "d510" = 1.5
  dimension "d513" = 1.5
  constraint horizontal L0
  constraint vertical L1
  constraint horizontal L2
  constraint vertical L3
  measures "d508" distance of L3 L4
  measures "d509" distance of L1 L5
  measures "d510" distance of L2 L6
  measures "d513" distance of L0 L7
extrude "Extrude62" cut sketch "Sketch46" against normal up to surface (4 mm away) bodies 3
ref_plane "Arbeitsebene17" through (0, 33.5, 0) normal (0, 1, 0) x (1, 0, 0)
sketch "Skizze47" plane through (0, 33.5, 0) normal (0, 1, 0) x (1, 0, 0)
  line L0 (-12, -25) -> (12, -25)
  line L1 (12, -25) -> (12, -16)
  line L2 (12, -16) -> (-12, -16)
  line L3 (-12, -16) -> (-12, -25)
  constraint horizontal L0
  constraint vertical L1
  constraint horizontal L2
  constraint vertical L3
extrude "Extrusion63" cut sketch "Skizze47" against normal up to surface (4 mm away) bodies 2
ref_plane "Arbeitsebene20" through (0, 14.75, 31.5) normal (0, 0, 1) x (1, 0, 0)
sketch "Skizze50" plane through (0, 14.75, 31.5) normal (0, 0, 1) x (1, 0, 0)
  line L0 (-12, -10) -> (12, -10)
  line L1 (12, -10) -> (12, -6)
  line L2 (12, -6) -> (-12, -6)
  line L3 (-12, -6) -> (-12, -10)
  constraint horizontal L0
  constraint vertical L1
  constraint horizontal L2
  constraint vertical L3
extrude "Extrusion66" cut sketch "Skizze50" against normal up to surface (4 mm away) bodies 3
sketch "Top" plane through (0, 33.5, 0) normal (0, 1, 0) x (-1, 0, 0) in component "DXF Export"
  circle A0 centre (0, 29.5) radius 0.8
  circle A1 centre (16.285, 0) radius 0.8
  circle A2 centre (-16.285, 0) radius 0.8
  circle A3 centre (0, -29.5) radius 0.8
  line L0 (-14.285, 18.5) -> (-18.285, 18.5)
  line L1 (-18.285, 18.5) -> (-18.285, -18.5)
  line L2 (-18.285, -18.5) -> (-14.285, -18.5)
  line L3 (-14.285, -18.5) -> (-14.285, -23)
  line L4 (-14.285, -23) -> (-18.285, -23)
  line L5 (-18.285, -23) -> (-18.285, -31.5)
  line L6 (-18.285, -31.5) -> (-9.785, -31.5)
  line L7 (-9.785, -31.5) -> (-9.785, -27.5)
  line L8 (-9.785, -27.5) -> (-5.285, -27.5)
  line L9 (-5.285, -27.5) -> (-5.285, -31.5)
  line L10 (-5.285, -31.5) -> (5.285, -31.5)
  line L11 (5.285, -31.5) -> (5.285, -27.5)
  line L12 (5.285, -27.5) -> (9.785, -27.5)
  line L13 (9.785, -27.5) -> (9.785, -31.5)
  line L14 (9.785, -31.5) -> (18.285, -31.5)
  line L15 (18.285, -31.5) -> (18.285, -23)
  line L16 (18.285, -23) -> (14.285, -23)
  line L17 (14.285, -23) -> (14.285, -18.5)
  line L18 (14.285, -18.5) -> (18.285, -18.5)
  line L19 (18.285, -18.5) -> (18.285, 18.5)
  line L20 (18.285, 18.5) -> (14.285, 18.5)
  line L21 (14.285, 18.5) -> (14.285, 23)
  line L22 (14.285, 23) -> (18.285, 23)
  line L23 (18.285, 23) -> (18.285, 31.5)
  line L24 (18.285, 31.5) -> (9.785, 31.5)
  line L25 (9.785, 31.5) -> (9.785, 27.5)
  line L26 (9.785, 27.5) -> (5.285, 27.5)
  line L27 (5.285, 27.5) -> (5.285, 31.5)
  line L28 (5.285, 31.5) -> (-5.285, 31.5)
  line L29 (-5.285, 31.5) -> (-5.285, 27.5)
  line L30 (-5.285, 27.5) -> (-9.785, 27.5)
  line L31 (-9.785, 27.5) -> (-9.785, 31.5)
  line L32 (-9.785, 31.5) -> (-18.285, 31.5)
  line L33 (-18.285, 31.5) -> (-18.285, 23)
  line L34 (-18.285, 23) -> (-14.285, 23)
  line L35 (-14.285, 23) -> (-14.285, 18.5)
  line L36 (12, 16) -> (-12, 16)
  line L37 (-12, 16) -> (-12, 25)
  line L38 (-12, 25) -> (12, 25)
  line L39 (12, 25) -> (12, 16)
sketch "Bottom" plane through (0, -4, 0) normal (0, -1, 0) x (1, 0, 0) in component "DXF Export"
  circle A0 centre (0, 29.5) radius 0.8
  circle A1 centre (-16.285, 0) radius 0.8
  circle A2 centre (0, -29.5) radius 0.8
  circle A3 centre (16.285, 0) radius 0.8
  line L0 (-14.285, 18.5) -> (-18.285, 18.5)
  line L1 (-18.285, 18.5) -> (-18.285, -18.5)
  line L2 (-18.285, -18.5) -> (-14.285, -18.5)
  line L3 (-14.285, -18.5) -> (-14.285, -23)
  line L4 (-14.285, -23) -> (-18.285, -23)
  line L5 (-18.285, -23) -> (-18.285, -31.5)
  line L6 (-18.285, -31.5) -> (-9.785, -31.5)
  line L7 (-9.785, -31.5) -> (-9.785, -27.5)
  line L8 (-9.785, -27.5) -> (-5.285, -27.5)
  line L9 (-5.285, -27.5) -> (-5.285, -31.5)
  line L10 (-5.285, -31.5) -> (5.285, -31.5)
  line L11 (5.285, -31.5) -> (5.285, -27.5)
  line L12 (5.285, -27.5) -> (9.785, -27.5)
  line L13 (9.785, -27.5) -> (9.785, -31.5)
  line L14 (9.785, -31.5) -> (18.285, -31.5)
  line L15 (18.285, -31.5) -> (18.285, -23)
  line L16 (18.285, -23) -> (14.285, -23)
  line L17 (14.285, -23) -> (14.285, -18.5)
  line L18 (14.285, -18.5) -> (18.285, -18.5)
  line L19 (18.285, -18.5) -> (18.285, 18.5)
  line L20 (18.285, 18.5) -> (14.285, 18.5)
  line L21 (14.285, 18.5) -> (14.285, 23)
  line L22 (14.285, 23) -> (18.285, 23)
  line L23 (18.285, 23) -> (18.285, 31.5)
  line L24 (18.285, 31.5) -> (9.785, 31.5)
  line L25 (9.785, 31.5) -> (9.785, 27.5)
  line L26 (9.785, 27.5) -> (5.285, 27.5)
  line L27 (5.285, 27.5) -> (5.285, 31.5)
  line L28 (5.285, 31.5) -> (-5.285, 31.5)
  line L29 (-5.285, 31.5) -> (-5.285, 27.5)
  line L30 (-5.285, 27.5) -> (-9.785, 27.5)
  line L31 (-9.785, 27.5) -> (-9.785, 31.5)
  line L32 (-9.785, 31.5) -> (-18.285, 31.5)
  line L33 (-18.285, 31.5) -> (-18.285, 23)
  line L34 (-18.285, 23) -> (-14.285, 23)
  line L35 (-14.285, 23) -> (-14.285, 18.5)
  line L36 (-7.9108, -14.1817) -> (8.0892, -14.1817)
  line L37 (8.0892, -14.1817) -> (8.0892, -23.1823)
  line L38 (8.0892, -23.1823) -> (-7.9108, -23.1823)
  line L39 (-7.9108, -23.1823) -> (-7.9108, -14.1817)
  line L40 (10.165, -24.52) -> (10.165, 24.32)
  line L41 (10.165, 24.32) -> (12.785, 24.32)
  line L42 (12.785, 24.32) -> (12.785, -24.52)
  line L43 (12.785, -24.52) -> (10.165, -24.52)
  line L44 (-12.785, 24.32) -> (-10.165, 24.32)
  line L45 (-10.165, 24.32) -> (-10.165, -24.52)
  line L46 (-10.165, -24.52) -> (-12.785, -24.52)
  line L47 (-12.785, -24.52) -> (-12.785, 24.32)
sketch "Front" plane through (0, 0, 31.5) normal (0, 0, 1) x (1, 0, 0) in component "DXF Export"
  line L0 (-12.35, 13) -> (-12.35, 17)
  line L1 (-12.35, 17) -> (-7.85, 17)
  line L2 (-7.85, 17) -> (-7.85, 13)
  line L3 (-7.85, 13) -> (-12.35, 13)
  circle A0 centre (16.285, 14.75) radius 0.8
  circle A1 centre (-16.285, 14.75) radius 0.8
  line L4 (-18.285, 20.5) -> (-18.285, 9)
  line L5 (-18.285, 9) -> (-14.285, 9)
  line L6 (-14.285, 9) -> (-14.285, 4.5)
  line L7 (-14.285, 4.5) -> (-18.285, 4.5)
  line L8 (-18.285, 4.5) -> (-18.285, 0)
  line L9 (-18.285, 0) -> (-9.785, 0)
  line L10 (-9.785, 0) -> (-9.785, -4)
  line L11 (-9.785, -4) -> (-5.285, -4)
  line L12 (-5.285, -4) -> (-5.285, 0)
  line L13 (-5.285, 0) -> (-0.8, 0)
  line L14 (-0.8, 0) -> (-0.8, 0.7)
  line L15 (-0.8, 0.7) -> (-1.6, 0.7)
  line L16 (-1.6, 0.7) -> (-1.6, 2.1)
  line L17 (-1.6, 2.1) -> (1.6, 2.1)
  line L18 (1.6, 2.1) -> (1.6, 0.7)
  line L19 (1.6, 0.7) -> (0.8, 0.7)
  line L20 (0.8, 0.7) -> (0.8, 0)
  line L21 (0.8, 0) -> (5.285, 0)
  line L22 (5.285, 0) -> (5.285, -4)
  line L23 (5.285, -4) -> (9.785, -4)
  line L24 (9.785, -4) -> (9.785, 0)
  line L25 (9.785, 0) -> (18.285, 0)
  line L26 (18.285, 0) -> (18.285, 4.5)
  line L27 (18.285, 4.5) -> (14.285, 4.5)
  line L28 (14.285, 4.5) -> (14.285, 9)
  line L29 (14.285, 9) -> (18.285, 9)
  line L30 (18.285, 9) -> (18.285, 20.5)
  line L31 (18.285, 29.5) -> (9.785, 29.5)
  line L32 (9.785, 29.5) -> (9.785, 33.5)
  line L33 (9.785, 33.5) -> (5.285, 33.5)
  line L34 (5.285, 33.5) -> (5.285, 29.5)
  line L35 (5.285, 29.5) -> (0.8, 29.5)
  line L36 (0.8, 29.5) -> (0.8, 28.8)
  line L37 (0.8, 28.8) -> (1.6, 28.8)
  line L38 (1.6, 28.8) -> (1.6, 27.4)
  line L39 (1.6, 27.4) -> (-1.6, 27.4)
  line L40 (-1.6, 27.4) -> (-1.6, 28.8)
  line L41 (-1.6, 28.8) -> (-0.8, 28.8)
  line L42 (-0.8, 28.8) -> (-0.8, 29.5)
  line L43 (-0.8, 29.5) -> (-5.285, 29.5)
  line L44 (-5.285, 29.5) -> (-5.285, 33.5)
  line L45 (-5.285, 33.5) -> (-9.785, 33.5)
  line L46 (-9.785, 33.5) -> (-9.785, 29.5)
  line L47 (-9.785, 29.5) -> (-18.285, 29.5)
  line L48 (-14.285, 25) -> (-14.285, 20.5)
  line L49 (-14.285, 20.5) -> (-18.285, 20.5)
  line L50 (18.285, 20.5) -> (14.285, 20.5)
  line L51 (14.285, 20.5) -> (14.285, 25)
  line L52 (14.285, 25) -> (18.285, 25)
  line L53 (18.285, 25) -> (18.285, 29.5)
  line L54 (-18.285, 29.5) -> (-18.285, 25)
  line L55 (-18.285, 25) -> (-14.285, 25)
  line L56 (-11.285, 25.9) -> (11.285, 25.9)
  line L57 (11.285, 25.9) -> (11.285, 18.5)
  line L58 (11.285, 18.5) -> (-11.285, 18.5)
  line L59 (-11.285, 18.5) -> (-11.285, 25.9)
  line L60 (-12, 8.75) -> (12, 8.75)
  line L61 (12, 8.75) -> (12, 4.75)
  line L62 (12, 4.75) -> (-12, 4.75)
  line L63 (-12, 4.75) -> (-12, 8.75)
sketch "Back" plane through (0, 0, -31.5) normal (0, 0, -1) x (-1, 0, 0) in component "DXF Export"
  line L0 (-12.35, 13) -> (-12.35, 17)
  line L1 (-12.35, 17) -> (-7.85, 17)
  line L2 (-7.85, 17) -> (-7.85, 13)
  line L3 (-7.85, 13) -> (-12.35, 13)
  circle A0 centre (16.285, 14.75) radius 0.8
  circle A1 centre (-16.285, 14.75) radius 0.8
  line L4 (0.8, 0.7) -> (0.8, 0)
  line L5 (0.8, 0) -> (5.285, 0)
  line L6 (5.285, 0) -> (5.285, -4)
  line L7 (5.285, -4) -> (9.785, -4)
  line L8 (9.785, -4) -> (9.785, 0)
  line L9 (9.785, 0) -> (18.285, 0)
  line L10 (18.285, 0) -> (18.285, 4.5)
  line L11 (18.285, 4.5) -> (14.285, 4.5)
  line L12 (14.285, 4.5) -> (14.285, 9)
  line L13 (14.285, 9) -> (18.285, 9)
  line L14 (18.285, 9) -> (18.285, 20.5)
  line L15 (18.285, 29.5) -> (9.785, 29.5)
  line L16 (9.785, 29.5) -> (9.785, 33.5)
  line L17 (9.785, 33.5) -> (5.285, 33.5)
  line L18 (5.285, 33.5) -> (5.285, 29.5)
  line L19 (5.285, 29.5) -> (0.8, 29.5)
  line L20 (0.8, 29.5) -> (0.8, 28.8)
  line L21 (0.8, 28.8) -> (1.6, 28.8)
  line L22 (1.6, 28.8) -> (1.6, 27.4)
  line L23 (1.6, 27.4) -> (-1.6, 27.4)
  line L24 (-1.6, 27.4) -> (-1.6, 28.8)
  line L25 (-1.6, 28.8) -> (-0.8, 28.8)
  line L26 (-0.8, 28.8) -> (-0.8, 29.5)
  line L27 (-0.8, 29.5) -> (-5.285, 29.5)
  line L28 (-5.285, 29.5) -> (-5.285, 33.5)
  line L29 (-5.285, 33.5) -> (-9.785, 33.5)
  line L30 (-9.785, 33.5) -> (-9.785, 29.5)
  line L31 (-9.785, 29.5) -> (-18.285, 29.5)
  line L32 (-18.285, 20.5) -> (-18.285, 9)
  line L33 (-18.285, 9) -> (-14.285, 9)
  line L34 (-14.285, 9) -> (-14.285, 4.5)
  line L35 (-14.285, 4.5) -> (-18.285, 4.5)
  line L36 (-18.285, 4.5) -> (-18.285, 0)
  line L37 (-18.285, 0) -> (-9.785, 0)
  line L38 (-9.785, 0) -> (-9.785, -4)
  line L39 (-9.785, -4) -> (-5.285, -4)
  line L40 (-5.285, -4) -> (-5.285, 0)
  line L41 (-5.285, 0) -> (-0.8, 0)
  line L42 (-0.8, 0) -> (-0.8, 0.7)
  line L43 (-0.8, 0.7) -> (-1.6, 0.7)
  line L44 (-1.6, 0.7) -> (-1.6, 2.1)
  line L45 (-1.6, 2.1) -> (1.6, 2.1)
  line L46 (1.6, 2.1) -> (1.6, 0.7)
  line L47 (1.6, 0.7) -> (0.8, 0.7)
  line L48 (18.285, 20.5) -> (14.285, 20.5)
  line L49 (14.285, 20.5) -> (14.285, 25)
  line L50 (14.285, 25) -> (18.285, 25)
  line L51 (18.285, 25) -> (18.285, 29.5)
  line L52 (-18.285, 29.5) -> (-18.285, 25)
  line L53 (-18.285, 25) -> (-14.285, 25)
  line L54 (-14.285, 25) -> (-14.285, 20.5)
  line L55 (-14.285, 20.5) -> (-18.285, 20.5)
sketch "Right" plane through (18.285, 0, 0) normal (1, 0, 0) x (0, 0, -1) in component "DXF Export"
  line L0 (-17.35, 13) -> (-17.35, 17)
  line L1 (-17.35, 17) -> (-12.85, 17)
  line L2 (-12.85, 17) -> (-12.85, 13)
  line L3 (-12.85, 13) -> (-17.35, 13)
  line L4 (-0.8, 29.5) -> (-18.5, 29.5)
  line L5 (-18.5, 29.5) -> (-18.5, 33.5)
  line L6 (-18.5, 33.5) -> (-23, 33.5)
  line L7 (-23, 33.5) -> (-23, 29.5)
  line L8 (-23, 29.5) -> (-27.5, 29.5)
  line L9 (-27.5, 29.5) -> (-27.5, 25)
  line L10 (-27.5, 15.55) -> (-26.8, 15.55)
  line L11 (-26.8, 15.55) -> (-26.8, 16.35)
  line L12 (-26.8, 16.35) -> (-25.4, 16.35)
  line L13 (-25.4, 16.35) -> (-25.4, 13.15)
  line L14 (-25.4, 13.15) -> (-26.8, 13.15)
  line L15 (-26.8, 13.15) -> (-26.8, 13.95)
  line L16 (-26.8, 13.95) -> (-27.5, 13.95)
  line L17 (-27.5, 13.95) -> (-27.5, 9)
  line L18 (-27.5, 9) -> (-31.5, 9)
  line L19 (-31.5, 9) -> (-31.5, 4.5)
  line L20 (-31.5, 4.5) -> (-27.5, 4.5)
  line L21 (-27.5, 4.5) -> (-27.5, 0)
  line L22 (-27.5, 0) -> (-23, 0)
  line L23 (-23, 0) -> (-23, -4)
  line L24 (-23, -4) -> (-18.5, -4)
  line L25 (-18.5, -4) -> (-18.5, 0)
  line L26 (-18.5, 0) -> (-0.8, 0)
  line L27 (-0.8, 0) -> (-0.8, 0.7)
  line L28 (-0.8, 0.7) -> (-1.6, 0.7)
  line L29 (-1.6, 0.7) -> (-1.6, 2.1)
  line L30 (-1.6, 2.1) -> (1.6, 2.1)
  line L31 (1.6, 2.1) -> (1.6, 0.7)
  line L32 (1.6, 0.7) -> (0.8, 0.7)
  line L33 (0.8, 0.7) -> (0.8, 0)
  line L34 (0.8, 0) -> (18.5, 0)
  line L35 (18.5, 0) -> (18.5, -4)
  line L36 (18.5, -4) -> (23, -4)
  line L37 (23, -4) -> (23, 0)
  line L38 (23, 0) -> (27.5, 0)
  line L39 (27.5, 0) -> (27.5, 4.5)
  line L40 (27.5, 4.5) -> (31.5, 4.5)
  line L41 (31.5, 4.5) -> (31.5, 9)
  line L42 (31.5, 9) -> (27.5, 9)
  line L43 (27.5, 9) -> (27.5, 13.95)
  line L44 (27.5, 13.95) -> (26.8, 13.95)
  line L45 (26.8, 13.95) -> (26.8, 13.15)
  line L46 (26.8, 13.15) -> (25.4, 13.15)
  line L47 (25.4, 13.15) -> (25.4, 16.35)
  line L48 (25.4, 16.35) -> (26.8, 16.35)
  line L49 (26.8, 16.35) -> (26.8, 15.55)
  line L50 (26.8, 15.55) -> (27.5, 15.55)
  line L51 (27.5, 15.55) -> (27.5, 20.5)
  line L52 (27.5, 29.5) -> (23, 29.5)
  line L53 (23, 29.5) -> (23, 33.5)
  line L54 (23, 33.5) -> (18.5, 33.5)
  line L55 (18.5, 33.5) -> (18.5, 29.5)
  line L56 (18.5, 29.5) -> (0.8, 29.5)
  line L57 (0.8, 29.5) -> (0.8, 28.8)
  line L58 (0.8, 28.8) -> (1.6, 28.8)
  line L59 (1.6, 28.8) -> (1.6, 27.4)
  line L60 (1.6, 27.4) -> (-1.6, 27.4)
  line L61 (-1.6, 27.4) -> (-1.6, 28.8)
  line L62 (-1.6, 28.8) -> (-0.8, 28.8)
  line L63 (-0.8, 28.8) -> (-0.8, 29.5)
  line L64 (-27.5, 25) -> (-31.5, 25)
  line L65 (-31.5, 25) -> (-31.5, 20.5)
  line L66 (-31.5, 20.5) -> (-27.5, 20.5)
  line L67 (-27.5, 20.5) -> (-27.5, 15.55)
  line L68 (27.5, 20.5) -> (31.5, 20.5)
  line L69 (31.5, 20.5) -> (31.5, 25)
  line L70 (31.5, 25) -> (27.5, 25)
  line L71 (27.5, 25) -> (27.5, 29.5)